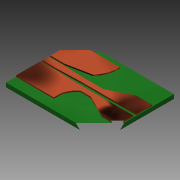
# Autodesk Inventor part: Balun
Saved by Autodesk Inventor 2014 (Build 180170000, 170)
## iProperties
Created: 2015-05-01
Part Number: Balun
Material: Generic
Document SubType Name: Modeling
Designer: Owner
Density: 1 g/cm^3
Appearance: Default
Author: Owner
Autodesk Inventor part; units mm, degrees
ref_plane "YZ Plane" through (0, 0, 0) normal (1, 0, 0) x (0, 1, 0)
ref_plane "XZ Plane" through (0, 0, 0) normal (0, 1, 0) x (-1, 0, 0)
ref_plane "XY Plane" through (0, 0, 0) normal (0, 0, 1) x (1, 0, 0)
sketch "Sketch1" plane through (0, 0, 0) normal (0, 1, 0) x (-1, 0, 0)
  line L0 (-20.6942, 15.5467) -> (17.4058, 15.5467)
  line L1 (17.4058, 15.5467) -> (17.4058, -14.4533)
  line L2 (17.4058, -14.4533) -> (-20.6942, -14.4533)
  line L3 (-20.6942, -14.4533) -> (-20.6942, 15.5467)
  point P0 (0, 0)
  dimension "d24" = 30
  dimension "d31" = 38.1
  constraints: 8 end point, 2 parallel, 1 horizontal, 1 perpendicular
  measures "d24" distance of L0.end L1.end
  measures "d31" distance of L0.start L0.end
extrude "Extrusion1" add sketch "Sketch1" along normal blind 1.65
sketch "Sketch2" plane through (0, 1.65, 0) normal (0, 1, 0) x (1, 0, 0)
  line L0 (20.6942, 14.4533) -> (-17.4058, 14.4533) projected
  line L1 (-17.4058, 14.4533) -> (-17.4058, -15.5467) projected
  line L2 (-13.4058, -0.8367) -> (-11.6058, -0.8367)
  line L3 (-11.6058, -0.8367) -> (-2.0058, -0.5567)
  line L4 (-2.0058, -0.5567) -> (5.1459, -0.5567)
  line L5 (-13.4058, 1.7633) -> (-13.5518, 1.7633)
  line L6 (-13.4058, -1.5267) -> (-11.6058, -1.5267)
  line L7 (5.1459, -3.7967) -> (1.0334, -3.7967)
  line L8 (-13.4058, 2.4533) -> (-11.6058, 2.4533)
  arc A0 (1.0334, -3.7967) -> (-2.0058, -8.5193) centre (6.5441, -10.6824) ccw
  line L9 (-13.4058, 2.4533) -> (-13.4058, 4.3733)
  line L10 (-13.4058, 4.3733) -> (-2.0058, 4.3733)
  line L11 (-13.4058, 1.7633) -> (-13.4058, -0.8367)
  line L12 (-13.4058, -1.5267) -> (-13.4058, -11.5267)
  line L13 (-13.4058, -11.5267) -> (-2.0058, -11.5267)
  line L14 (-2.0058, -11.5267) -> (-2.0058, -8.5193)
  line L15 (5.1459, -3.7967) -> (5.1459, -1.8067)
  line L16 (5.1459, -0.5567) -> (5.1459, 1.4333)
  line L17 (-2.0058, -1.8067) -> (5.1459, -1.8067)
  line L18 (-13.4058, 1.7633) -> (-11.6058, 1.7633)
  line L19 (-11.6058, 1.7633) -> (-2.0058, 1.4333)
  line L20 (-2.0058, 1.4333) -> (5.1459, 1.4333)
  line L21 (-11.6058, 2.4533) -> (-2.0058, 4.3733)
  line L22 (-11.6058, -1.5267) -> (-2.0058, -1.8067)
  line L23 (-13.4058, 4.3733) -> (-13.4058, 12.4533)
  line L24 (-13.4058, 12.4533) -> (0.7657, 12.4533)
  arc A1 (-2.0058, 4.3733) -> (0.7657, 12.4533) centre (-10.6902, 11.8674) ccw
  line L25 (-13.4058, 12.4533) -> (-17.4058, 12.4533)
  line L26 (-17.4058, 12.4533) -> (-17.4058, 2.4533)
  line L27 (-17.4058, 2.4533) -> (-13.4058, 2.4533)
  line L28 (-13.4058, 2.4533) -> (-13.4058, 12.4533)
  line L29 (-13.4058, -1.5267) -> (-17.4058, -1.5267)
  line L30 (-17.4058, -1.5267) -> (-17.4058, -11.5267)
  line L31 (-17.4058, -11.5267) -> (-13.4058, -11.5267)
  line L32 (-13.4058, -11.5267) -> (-13.4058, -1.5267)
  line L33 (-13.4058, -0.8367) -> (-17.4058, -0.8367)
  line L34 (-17.4058, -0.8367) -> (-17.4058, 1.7633)
  line L35 (-17.4058, 1.7633) -> (-13.4058, 1.7633)
  line L36 (-13.4058, 1.7633) -> (-13.4058, -0.8367)
  line L37 (5.1489, 1.4333) -> (5.1459, -0.5567)
  line L38 (5.1459, -2.1721) -> (5.1459, -3.7967)
  line L39 (14.0359, -0.5567) -> (14.0359, 5.7933)
  line L40 (14.0359, 5.7933) -> (5.1489, 1.4333)
  line L41 (5.1459, -1.8067) -> (14.0359, -1.8067)
  line L42 (14.0359, -1.8067) -> (14.0359, -8.1567)
  line L43 (14.0359, -8.1567) -> (5.1459, -3.7967)
  line L44 (5.1459, -0.5567) -> (14.0359, -0.5567)
  line L45 (14.0359, 5.7933) -> (20.3859, 5.7933)
  line L46 (20.3859, 5.7933) -> (20.3859, -0.5567)
  line L47 (20.3859, -0.5567) -> (14.0359, -0.5567)
  line L48 (14.0359, -0.5567) -> (14.0359, 5.7933)
  line L49 (14.0359, -8.1567) -> (20.3859, -8.1567)
  line L50 (20.3859, -8.1567) -> (20.3859, -1.8067)
  line L51 (20.3859, -1.8067) -> (14.0359, -1.8067)
  line L52 (14.0359, -1.8067) -> (14.0359, -8.1567)
  point P0 (0, 0)
  dimension "d2" = 2.6
  dimension "d3" = 0.69
  dimension "d4" = 0.69
  dimension "d5" = 1.99
  dimension "d7" = 1.8
  dimension "d8" = 1.8
  dimension "d10" = 10
  dimension "d11" = 1.8
  dimension "d12" = 1.25
  dimension "d14" = 1.8
  dimension "d15" = 0.28
  dimension "d16" = 1.99
  dimension "d17" = 9.6
  dimension "d18" = 9.6
  dimension "d19" = 9.6
  dimension "d20" = 9.6
  dimension "d21" = 2.94
  dimension "d22" = 0
  dimension "d23" = 10
  dimension "d25" = 4
  dimension "d27" = 0
  dimension "d28" = 2
  dimension "d32" = 6.35
  dimension "d33" = 6.35
  dimension "d34" = 8.89
  dimension "d35" = 6.35
  constraints: 102 end point, 18 perpendicular, 16 parallel, 12 collinear, 5 horizontal, 4 point on circle, 2 centre point
  measures "d2" distance of L5.start L2.start
  measures "d3" distance between parallel lines of L6 L2
  measures "d4" distance between parallel lines of L8 L5
  measures "d5" distance of L7.start L15.end
  measures "d7" distance of L2.start L2.end
  measures "d8" distance of L8.start L8.end
  measures "d10" distance of L6.start L12.end
  measures "d11" distance of L6.start L6.end
  measures "d12" distance between parallel lines of L17 L4
  measures "d14" distance of L5.start L18.end
  measures "d15" distance between parallel lines of L17 L6
  measures "d16" distance of L4.end L16.end
  measures "d17" horizontal distance of L17.start L6.end
  measures "d18" horizontal distance of L3.end L2.end
  measures "d19" horizontal distance of L19.end L18.end
  measures "d20" horizontal distance of L10.end L8.end
  measures "d21" distance from line of L20 L10.end
  measures "d22" distance from line of L14 L17.start
  measures "d23" distance between parallel lines of L24 L8
  measures "d25" distance of L23.end L25.end
  measures "d27" distance between parallel lines of L1 L26
  measures "d28" distance between parallel lines of L0 L24
  measures "d32" distance of L39.start L39.end
  measures "d33" distance of L41.end L42.end
  measures "d34" distance between parallel lines of L39 L16
  measures "d35" distance of L39.end L45.end
extrude "Extrusion2" add sketch "Sketch2" along normal blind 0.5
body "Solid1"
